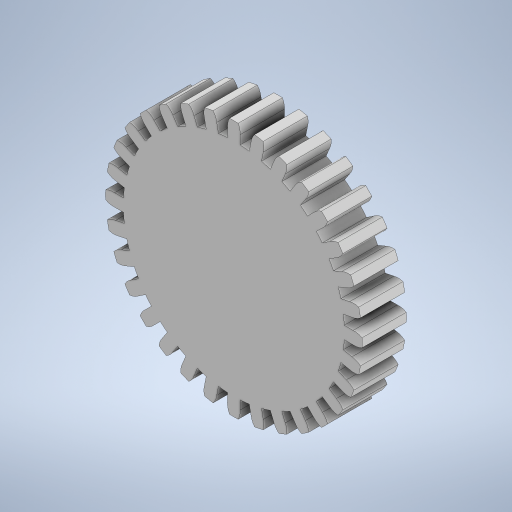
# Autodesk Inventor part: Geear
Saved by Autodesk Inventor 2024 (Build 280153000, 153)
## iProperties
Created: 2024-09-11
Part Number: Geear
Material: Generic
Document SubType Name: Modeling
Designer: srira
Density: 1 g/cm^3
Appearance: Default
Author: srira
Autodesk Inventor part; units mm, degrees
ref_plane "YZ Plane" through (0, 0, 0) normal (1, 0, 0) x (0, 1, 0)
ref_plane "XZ Plane" through (0, 0, 0) normal (0, 1, 0) x (-1, 0, 0)
ref_plane "XY Plane" through (0, 0, 0) normal (0, 0, 1) x (1, 0, 0)
sketch "Sketch1" plane through (0, 0, 0) normal (0, 0, 1) x (1, 0, 0)
  line L0 (0, 0) -> (-1.4131, 26.963) construction
  line L1 (0, 0) -> (27, 0) construction
  line L2 (0, 0) -> (1.4131, 26.963) construction
  line L3 (0, 0) -> (27, 0) construction
  line L4 (-1.4131, 26.963) -> (-1.4131, 24.463)
  line L5 (-1.4131, 26.963) -> (1.0869, 26.963) construction
  line L6 (1.4131, 26.963) -> (1.4131, 24.463)
  line L7 (1.4131, 26.963) -> (3.9131, 26.963) construction
  arc A0 (-0.7919, 29.2812) -> (-1.4131, 26.963) centre (2.0733, 27.2711) ccw
  line L8 (-1.4131, 26.963) -> (-0.7919, 29.2812) construction
  line L9 (-1.4131, 26.963) -> (0.9869, 26.963) construction
  arc A1 (1.4131, 26.963) -> (0.7919, 29.2812) centre (-2.0733, 27.2711) ccw
  line L10 (1.4131, 26.963) -> (0.7919, 29.2812) construction
  line L11 (1.4131, 26.963) -> (3.8131, 26.963) construction
  line L12 (-6.6461, 26.1692) -> (-6.1584, 23.7173)
  arc A2 (-6.4892, 28.5641) -> (-6.6461, 26.1692) centre (-3.2868, 27.1516) ccw
  arc A3 (-3.8743, 26.7206) -> (-4.9358, 28.8731) centre (-7.3538, 26.3427) ccw
  line L13 (-3.8743, 26.7206) -> (-3.3866, 24.2686)
  line L14 (-11.6238, 24.3698) -> (-10.6671, 22.0601)
  arc A4 (-11.9371, 26.7493) -> (-11.6238, 24.3698) centre (-8.5207, 25.9887) ccw
  arc A5 (-9.0128, 25.4513) -> (-10.4738, 27.3554) centre (-12.3517, 24.4018) ccw
  line L15 (-9.0128, 25.4513) -> (-8.0561, 23.1416)
  line L16 (-16.1548, 21.6339) -> (-14.7658, 19.5552)
  arc A6 (-16.9262, 23.9065) -> (-16.1548, 21.6339) centre (-13.4271, 23.827) ccw
  arc A7 (-13.8049, 23.204) -> (-15.6093, 24.7864) centre (-16.875, 21.5232) ccw
  line L17 (-13.8049, 23.204) -> (-12.416, 21.1253)
  line L18 (-20.0649, 18.0665) -> (-18.2971, 16.2988)
  arc A8 (-21.2649, 20.145) -> (-20.0649, 18.0665) centre (-17.8175, 20.7497) ccw
  arc A9 (-18.0665, 20.0649) -> (-20.145, 21.2649) centre (-20.7497, 17.8175) ccw
  line L19 (-18.0665, 20.0649) -> (-16.2988, 18.2971)
  line L20 (-23.204, 13.8049) -> (-21.1253, 12.416)
  arc A10 (-24.7864, 15.6093) -> (-23.204, 13.8049) centre (-21.5232, 16.875) ccw
  arc A11 (-21.6339, 16.1548) -> (-23.9065, 16.9262) centre (-23.827, 13.4271) ccw
  line L21 (-21.6339, 16.1548) -> (-19.5552, 14.7658)
  line L22 (-25.4513, 9.0128) -> (-23.1416, 8.0561)
  arc A12 (-27.3554, 10.4738) -> (-25.4513, 9.0128) centre (-24.4018, 12.3517) ccw
  arc A13 (-24.3698, 11.6238) -> (-26.7493, 11.9371) centre (-25.9887, 8.5207) ccw
  line L23 (-24.3698, 11.6238) -> (-22.0601, 10.6671)
  line L24 (-26.7206, 3.8743) -> (-24.2686, 3.3866)
  arc A14 (-28.8731, 4.9358) -> (-26.7206, 3.8743) centre (-26.3427, 7.3538) ccw
  arc A15 (-26.1692, 6.6461) -> (-28.5641, 6.4892) centre (-27.1516, 3.2868) ccw
  line L25 (-26.1692, 6.6461) -> (-23.7173, 6.1584)
  line L26 (-26.963, -1.4131) -> (-24.463, -1.4131)
  arc A16 (-29.2812, -0.7919) -> (-26.963, -1.4131) centre (-27.2711, 2.0733) ccw
  arc A17 (-26.963, 1.4131) -> (-29.2812, 0.7919) centre (-27.2711, -2.0733) ccw
  line L27 (-26.963, 1.4131) -> (-24.463, 1.4131)
  line L28 (-26.1692, -6.6461) -> (-23.7173, -6.1584)
  arc A18 (-28.5641, -6.4892) -> (-26.1692, -6.6461) centre (-27.1516, -3.2868) ccw
  arc A19 (-26.7206, -3.8743) -> (-28.8731, -4.9358) centre (-26.3427, -7.3538) ccw
  line L29 (-26.7206, -3.8743) -> (-24.2686, -3.3866)
  line L30 (-24.3698, -11.6238) -> (-22.0601, -10.6671)
  arc A20 (-26.7493, -11.9371) -> (-24.3698, -11.6238) centre (-25.9887, -8.5207) ccw
  arc A21 (-25.4513, -9.0128) -> (-27.3554, -10.4738) centre (-24.4018, -12.3517) ccw
  line L31 (-25.4513, -9.0128) -> (-23.1416, -8.0561)
  line L32 (-21.6339, -16.1548) -> (-19.5552, -14.7658)
  arc A22 (-23.9065, -16.9262) -> (-21.6339, -16.1548) centre (-23.827, -13.4271) ccw
  arc A23 (-23.204, -13.8049) -> (-24.7864, -15.6093) centre (-21.5232, -16.875) ccw
  line L33 (-23.204, -13.8049) -> (-21.1253, -12.416)
  line L34 (-18.0665, -20.0649) -> (-16.2988, -18.2971)
  arc A24 (-20.145, -21.2649) -> (-18.0665, -20.0649) centre (-20.7497, -17.8175) ccw
  arc A25 (-20.0649, -18.0665) -> (-21.2649, -20.145) centre (-17.8175, -20.7497) ccw
  line L35 (-20.0649, -18.0665) -> (-18.2971, -16.2988)
  line L36 (-13.8049, -23.204) -> (-12.416, -21.1253)
  arc A26 (-15.6093, -24.7864) -> (-13.8049, -23.204) centre (-16.875, -21.5232) ccw
  arc A27 (-16.1548, -21.6339) -> (-16.9262, -23.9065) centre (-13.4271, -23.827) ccw
  line L37 (-16.1548, -21.6339) -> (-14.7658, -19.5552)
  line L38 (-9.0128, -25.4513) -> (-8.0561, -23.1416)
  arc A28 (-10.4738, -27.3554) -> (-9.0128, -25.4513) centre (-12.3517, -24.4018) ccw
  arc A29 (-11.6238, -24.3698) -> (-11.9371, -26.7493) centre (-8.5207, -25.9887) ccw
  line L39 (-11.6238, -24.3698) -> (-10.6671, -22.0601)
  line L40 (-3.8743, -26.7206) -> (-3.3866, -24.2686)
  arc A30 (-4.9358, -28.8731) -> (-3.8743, -26.7206) centre (-7.3538, -26.3427) ccw
  arc A31 (-6.6461, -26.1692) -> (-6.4892, -28.5641) centre (-3.2868, -27.1516) ccw
  line L41 (-6.6461, -26.1692) -> (-6.1584, -23.7173)
  line L42 (1.4131, -26.963) -> (1.4131, -24.463)
  arc A32 (0.7919, -29.2812) -> (1.4131, -26.963) centre (-2.0733, -27.2711) ccw
  arc A33 (-1.4131, -26.963) -> (-0.7919, -29.2812) centre (2.0733, -27.2711) ccw
  line L43 (-1.4131, -26.963) -> (-1.4131, -24.463)
  line L44 (6.6461, -26.1692) -> (6.1584, -23.7173)
  arc A34 (6.4892, -28.5641) -> (6.6461, -26.1692) centre (3.2868, -27.1516) ccw
  arc A35 (3.8743, -26.7206) -> (4.9358, -28.8731) centre (7.3538, -26.3427) ccw
  line L45 (3.8743, -26.7206) -> (3.3866, -24.2686)
  line L46 (11.6238, -24.3698) -> (10.6671, -22.0601)
  arc A36 (11.9371, -26.7493) -> (11.6238, -24.3698) centre (8.5207, -25.9887) ccw
  arc A37 (9.0128, -25.4513) -> (10.4738, -27.3554) centre (12.3517, -24.4018) ccw
  line L47 (9.0128, -25.4513) -> (8.0561, -23.1416)
  line L48 (16.1548, -21.6339) -> (14.7658, -19.5552)
  arc A38 (16.9262, -23.9065) -> (16.1548, -21.6339) centre (13.4271, -23.827) ccw
  arc A39 (13.8049, -23.204) -> (15.6093, -24.7864) centre (16.875, -21.5232) ccw
  line L49 (13.8049, -23.204) -> (12.416, -21.1253)
  line L50 (20.0649, -18.0665) -> (18.2971, -16.2988)
  arc A40 (21.2649, -20.145) -> (20.0649, -18.0665) centre (17.8175, -20.7497) ccw
  arc A41 (18.0665, -20.0649) -> (20.145, -21.2649) centre (20.7497, -17.8175) ccw
  line L51 (18.0665, -20.0649) -> (16.2988, -18.2971)
  line L52 (23.204, -13.8049) -> (21.1253, -12.416)
  arc A42 (24.7864, -15.6093) -> (23.204, -13.8049) centre (21.5232, -16.875) ccw
  arc A43 (21.6339, -16.1548) -> (23.9065, -16.9262) centre (23.827, -13.4271) ccw
  line L53 (21.6339, -16.1548) -> (19.5552, -14.7658)
  line L54 (25.4513, -9.0128) -> (23.1416, -8.0561)
  arc A44 (27.3554, -10.4738) -> (25.4513, -9.0128) centre (24.4018, -12.3517) ccw
  arc A45 (24.3698, -11.6238) -> (26.7493, -11.9371) centre (25.9887, -8.5207) ccw
  line L55 (24.3698, -11.6238) -> (22.0601, -10.6671)
  line L56 (26.7206, -3.8743) -> (24.2686, -3.3866)
  arc A46 (28.8731, -4.9358) -> (26.7206, -3.8743) centre (26.3427, -7.3538) ccw
  arc A47 (26.1692, -6.6461) -> (28.5641, -6.4892) centre (27.1516, -3.2868) ccw
  line L57 (26.1692, -6.6461) -> (23.7173, -6.1584)
  line L58 (26.963, 1.4131) -> (24.463, 1.4131)
  arc A48 (29.2812, 0.7919) -> (26.963, 1.4131) centre (27.2711, -2.0733) ccw
  arc A49 (26.963, -1.4131) -> (29.2812, -0.7919) centre (27.2711, 2.0733) ccw
  line L59 (26.963, -1.4131) -> (24.463, -1.4131)
  line L60 (26.1692, 6.6461) -> (23.7173, 6.1584)
  arc A50 (28.5641, 6.4892) -> (26.1692, 6.6461) centre (27.1516, 3.2868) ccw
  arc A51 (26.7206, 3.8743) -> (28.8731, 4.9358) centre (26.3427, 7.3538) ccw
  line L61 (26.7206, 3.8743) -> (24.2686, 3.3866)
  line L62 (24.3698, 11.6238) -> (22.0601, 10.6671)
  arc A52 (26.7493, 11.9371) -> (24.3698, 11.6238) centre (25.9887, 8.5207) ccw
  arc A53 (25.4513, 9.0128) -> (27.3554, 10.4738) centre (24.4018, 12.3517) ccw
  line L63 (25.4513, 9.0128) -> (23.1416, 8.0561)
  line L64 (21.6339, 16.1548) -> (19.5552, 14.7658)
  arc A54 (23.9065, 16.9262) -> (21.6339, 16.1548) centre (23.827, 13.4271) ccw
  arc A55 (23.204, 13.8049) -> (24.7864, 15.6093) centre (21.5232, 16.875) ccw
  line L65 (23.204, 13.8049) -> (21.1253, 12.416)
  line L66 (18.0665, 20.0649) -> (16.2988, 18.2971)
  arc A56 (20.145, 21.2649) -> (18.0665, 20.0649) centre (20.7497, 17.8175) ccw
  arc A57 (20.0649, 18.0665) -> (21.2649, 20.145) centre (17.8175, 20.7497) ccw
  line L67 (20.0649, 18.0665) -> (18.2971, 16.2988)
  line L68 (13.8049, 23.204) -> (12.416, 21.1253)
  arc A58 (15.6093, 24.7864) -> (13.8049, 23.204) centre (16.875, 21.5232) ccw
  arc A59 (16.1548, 21.6339) -> (16.9262, 23.9065) centre (13.4271, 23.827) ccw
  line L69 (16.1548, 21.6339) -> (14.7658, 19.5552)
  line L70 (9.0128, 25.4513) -> (8.0561, 23.1416)
  arc A60 (10.4738, 27.3554) -> (9.0128, 25.4513) centre (12.3517, 24.4018) ccw
  arc A61 (11.6238, 24.3698) -> (11.9371, 26.7493) centre (8.5207, 25.9887) ccw
  line L71 (11.6238, 24.3698) -> (10.6671, 22.0601)
  line L72 (3.8743, 26.7206) -> (3.3866, 24.2686)
  arc A62 (4.9358, 28.8731) -> (3.8743, 26.7206) centre (7.3538, 26.3427) ccw
  arc A63 (6.6461, 26.1692) -> (6.4892, 28.5641) centre (3.2868, 27.1516) ccw
  line L73 (6.6461, 26.1692) -> (6.1584, 23.7173)
  arc A64 (3.4835, 24.7561) -> (1.3084, 24.9657) centre (0, 0) ccw
  arc A65 (8.2463, 23.6008) -> (6.2554, 24.2048) centre (0, 0) ccw
  arc A66 (12.6921, 21.5386) -> (10.8573, 22.5193) centre (0, 0) ccw
  arc A67 (16.6502, 18.6486) -> (15.042, 19.9684) centre (0, 0) ccw
  arc A68 (19.9684, 15.042) -> (18.6486, 16.6502) centre (0, 0) ccw
  arc A69 (22.5193, 10.8573) -> (21.5386, 12.6921) centre (0, 0) ccw
  arc A70 (27, 0) -> (26.963, 1.4131) centre (0, 0) ccw
  arc A71 (24.2048, 6.2554) -> (23.6008, 8.2463) centre (0, 0) ccw
  arc A72 (24.96, 1.4131) -> (24.7561, 3.4835) centre (0, 0) ccw
  arc A73 (24.7561, -3.4835) -> (25, 0) centre (0, 0) ccw
  arc A74 (23.6008, -8.2463) -> (24.2048, -6.2554) centre (0, 0) ccw
  arc A75 (21.5386, -12.6921) -> (22.5193, -10.8573) centre (0, 0) ccw
  arc A76 (18.6486, -16.6502) -> (19.9684, -15.042) centre (0, 0) ccw
  arc A77 (15.042, -19.9684) -> (16.6502, -18.6486) centre (0, 0) ccw
  arc A78 (10.8573, -22.5193) -> (12.6921, -21.5386) centre (0, 0) ccw
  arc A79 (6.2554, -24.2048) -> (8.2463, -23.6008) centre (0, 0) ccw
  arc A80 (1.4131, -24.96) -> (3.4835, -24.7561) centre (0, 0) ccw
  arc A81 (-3.4835, -24.7561) -> (-1.4131, -24.96) centre (0, 0) ccw
  arc A82 (-8.2463, -23.6008) -> (-6.2554, -24.2048) centre (0, 0) ccw
  arc A83 (-12.6921, -21.5386) -> (-10.8573, -22.5193) centre (0, 0) ccw
  arc A84 (-16.6502, -18.6486) -> (-15.042, -19.9684) centre (0, 0) ccw
  arc A85 (-19.9684, -15.042) -> (-18.6486, -16.6502) centre (0, 0) ccw
  arc A86 (-22.5193, -10.8573) -> (-21.5386, -12.6921) centre (0, 0) ccw
  arc A87 (-24.2048, -6.2554) -> (-23.6008, -8.2463) centre (0, 0) ccw
  arc A88 (-24.96, -1.4131) -> (-24.7561, -3.4835) centre (0, 0) ccw
  arc A89 (-24.7561, 3.4835) -> (-24.96, 1.4131) centre (0, 0) ccw
  arc A90 (-23.6008, 8.2463) -> (-24.2048, 6.2554) centre (0, 0) ccw
  arc A91 (-21.5386, 12.6921) -> (-22.5193, 10.8573) centre (0, 0) ccw
  arc A92 (-18.6486, 16.6502) -> (-19.9684, 15.042) centre (0, 0) ccw
  arc A93 (-15.042, 19.9684) -> (-16.6502, 18.6486) centre (0, 0) ccw
  arc A94 (-10.8573, 22.5193) -> (-12.6921, 21.5386) centre (0, 0) ccw
  arc A95 (-1.3084, 24.9657) -> (-3.4835, 24.7561) centre (0, 0) ccw
  arc A96 (-6.2554, 24.2048) -> (-8.2463, 23.6008) centre (0, 0) ccw
  arc A97 (-1.4131, 26.963) -> (-3.8743, 26.7206) centre (0, 0) ccw
  arc A98 (-27.152, -10.1868) -> (-26.4025, -11.9962) centre (0, 0) ccw
  arc A99 (-28.6176, -4.694) -> (-28.2355, -6.6148) centre (0, 0) ccw
  arc A100 (-28.9835, 0.9792) -> (-28.9835, -0.9792) centre (0, 0) ccw
  arc A101 (-28.2355, 6.6148) -> (-28.6176, 4.694) centre (0, 0) ccw
  arc A102 (-26.4025, 11.9962) -> (-27.152, 10.1868) centre (0, 0) ccw
  arc A103 (-23.5549, 16.9165) -> (-24.6429, 15.2882) centre (0, 0) ccw
  arc A104 (-19.802, 21.1868) -> (-21.1868, 19.802) centre (0, 0) ccw
  arc A105 (-15.2882, 24.6429) -> (-16.9165, 23.5549) centre (0, 0) ccw
  arc A106 (-10.1868, 27.152) -> (-11.9962, 26.4025) centre (0, 0) ccw
  arc A107 (-4.694, 28.6176) -> (-6.6148, 28.2355) centre (0, 0) ccw
  arc A108 (0.9792, 28.9835) -> (-0.9792, 28.9835) centre (0, 0) ccw
  arc A109 (6.6148, 28.2355) -> (4.694, 28.6176) centre (0, 0) ccw
  arc A110 (11.9962, 26.4025) -> (10.1868, 27.152) centre (0, 0) ccw
  arc A111 (16.9165, 23.5549) -> (15.2882, 24.6429) centre (0, 0) ccw
  arc A112 (21.1868, 19.802) -> (19.802, 21.1868) centre (0, 0) ccw
  arc A113 (24.6429, 15.2882) -> (23.5549, 16.9165) centre (0, 0) ccw
  arc A114 (27.152, 10.1868) -> (26.4025, 11.9962) centre (0, 0) ccw
  arc A115 (28.6176, 4.694) -> (28.2355, 6.6148) centre (0, 0) ccw
  arc A116 (28.9835, -0.9792) -> (28.9835, 0.9792) centre (0, 0) ccw
  arc A117 (28.2355, -6.6148) -> (28.6176, -4.694) centre (0, 0) ccw
  arc A118 (26.4025, -11.9962) -> (27.152, -10.1868) centre (0, 0) ccw
  arc A119 (23.5549, -16.9165) -> (24.6429, -15.2882) centre (0, 0) ccw
  arc A120 (19.802, -21.1868) -> (21.1868, -19.802) centre (0, 0) ccw
  arc A121 (15.2882, -24.6429) -> (16.9165, -23.5549) centre (0, 0) ccw
  arc A122 (10.1868, -27.152) -> (11.9962, -26.4025) centre (0, 0) ccw
  arc A123 (4.694, -28.6176) -> (6.6148, -28.2355) centre (0, 0) ccw
  arc A124 (-0.9792, -28.9835) -> (0.9792, -28.9835) centre (0, 0) ccw
  arc A125 (-6.6148, -28.2355) -> (-4.694, -28.6176) centre (0, 0) ccw
  arc A126 (-11.9962, -26.4025) -> (-10.1868, -27.152) centre (0, 0) ccw
  arc A127 (-16.9165, -23.5549) -> (-15.2882, -24.6429) centre (0, 0) ccw
  arc A128 (-24.6429, -15.2882) -> (-23.5549, -16.9165) centre (0, 0) ccw
  arc A129 (-21.1868, -19.802) -> (-19.802, -21.1868) centre (0, 0) ccw
  point P0 (24.96, -1.4131)
  point P1 (1.4131, 24.96)
  point P2 (-1.4131, 24.96)
  dimension "d4" = 87
  dimension "d3" = 93
  dimension "d5" = 90
  dimension "d6" = 2.5
  dimension "d7" = 2.5
  dimension "d8" = 90
  dimension "d9" = 2.4
  dimension "d10" = 75
  dimension "d11" = 3.5
  dimension "d12" = 2.4
  dimension "d13" = 105
  dimension "d14" = 3.5
  dimension "d17" = 360
  constraints: 196 point on circle, 141 end point, 66 centre point, 61 point on line, 8 horizontal, 3 horizontal alignment, 2 equal length, 2 vertical alignment, 1 vertical, 584 other
  measures "d5" angle of L4 L5
  measures "d6" distance of L4.start L4.end
  measures "d7" distance of L6.start L6.end
  measures "d8" angle of L6 L7
  measures "d9" distance of L4.start L8.end
  measures "d10" angle of L9 L8
  measures "d11" radius of A0
  measures "d12" distance of L6.start L10.end
  measures "d13" angle of L11 L10
  measures "d14" radius of A1
extrude "Extrusion1" add sketch "Sketch1" along normal blind 10 contours A0 A108 A1 L6 A64 L72 A62 A109 A63 L73 A65 L70 A60 A110 A61 L71 A66 L68 A58 A111 A59 L69 A67 L66 A56 A112 A57 L67 A68 L64 A54 A113 A55 L65 A69 L62 A52 A114 A53 L63 A71 L60 A50 A115 A51 L61 A72 L58 A48 A116 A49 L59 A73 L56 A46 A117 A47 L57 A74 L54 A44 A118 A45 L55 A75 L52 A42 A119 A43 L53 A76 L50 A40 A120 A41 L51 A77 L48 A38 A121 A39 L49 A78 L46 A36 A122 A37 L47 A79 L44 A34 A123 A35 L45 A80 L42 A32 A124 A33 L43 A81 L40 A30 A125 A31 L41 A82 L38 A28 A126 A29 L39 A83 L36 A26 A127 A27 L37 A84 L34 A24 A129 A25 L35 A85 L32 A22 A128 A23 L33 A86 L30 A20 A98 A21 L31 A87 L28 A18 A99 A19 L29 A88 L26 A16 A100 A17 L27 A89 L24 A14 A101 A15 L25 A90 L22 A12 A102 A13 L23 A91 L20 A10 A103 A11 L21 A92 L18 A8 A104 A9 L19 A93 L16 A6 A105 A7 L17 A94 L14 A4 A106 A5 L15 A96 L12 A2 A107 A3 L13 A95 L4
body "Solid1"
